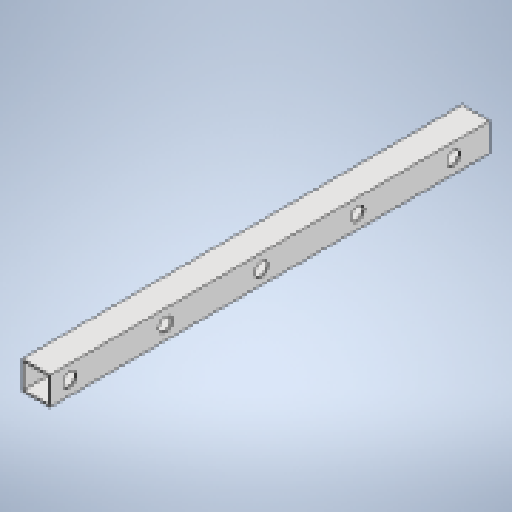
# Autodesk Inventor part: ANP 1434 FDS WAY tube4
Saved by Autodesk Inventor 2025.3 (Build 293356030, 356C)
## iProperties
Created: 2025-06-24
Part Number: ANP 1434 FDS WAY tube4
Material: Stainless Steel
Document SubType Name: Modeling
Designer: admin
Mass: 1762.25 g
Surface Area: 2283.33 cm^2
Volume: 220.281 cm^3
Density: 8 g/cm^3
Sheet Metal Rule: AISI304 2mm Die16
Sheet Metal Width: 0.000 mm
Sheet Metal Length: 0.000 mm
Sheet Metal Area: 0.000 mm^2
Appearance: Default
Stock Number: 30x30
Author: user
Autodesk Inventor part; units mm, degrees
ref_plane "YZ Plane" through (0, 0, 0) normal (1, 0, 0) x (0, 1, 0)
ref_plane "XZ Plane" through (0, 0, 0) normal (0, 1, 0) x (-1, 0, 0)
ref_plane "XY Plane" through (0, 0, 0) normal (0, 0, 1) x (1, 0, 0)
sketch "Sketch9" plane through (0, 0, 0) normal (0, 1, 0) x (-1, 0, 0)
  line L0 (17.5, 17.5) -> (-17.5, 17.5)
  line L1 (-17.5, 17.5) -> (-17.5, -17.5)
  line L2 (-17.5, -17.5) -> (17.5, -17.5)
  line L3 (17.5, -17.5) -> (17.5, 17.5)
  line L4 (17.5, 17.5) -> (-17.5, -17.5) construction
  line L5 (-17.5, 17.5) -> (17.5, -17.5) construction
  line L6 (-15.5, 15.5) -> (15.5, 15.5)
  line L7 (15.5, 15.5) -> (15.5, -15.5)
  line L8 (15.5, -15.5) -> (-15.5, -15.5)
  line L9 (-15.5, -15.5) -> (-15.5, 15.5)
  point P0 (0, 0)
  dimension "d172" = 35
  dimension "d173" = 35
  dimension "d174" = 2
  constraints: 20 end point, 4 parallel, 2 midpoint, 2 perpendicular, 1 horizontal, 3 other
  measures "d172" distance of L2.end L1.end
  measures "d173" distance of L0.end L1.end
  measures "d174" distance between parallel lines of L0 L6
extrude "Extrusion3" add sketch "Sketch9" against normal blind 550
sketch "Sketch10" plane through (0, 0, 0) normal (1, 0, 0) x (0, 1, 0)
  line L0 (0, 17.5) -> (0, -17.5) construction
  line L1 (0, 17.5) -> (-550, 17.5) construction
  line L2 (-550, -17.5) -> (-550, 17.5) construction
  line L3 (0, -17.5) -> (-550, -17.5) construction
  line L4 (-534, 8.5) -> (-517, 8.5)
  line L5 (-517, 8.5) -> (-517, -8.5)
  line L6 (-517, -8.5) -> (-534, -8.5)
  line L7 (-534, -8.5) -> (-534, 8.5)
  line L8 (-534, 8.5) -> (-517, -8.5) construction
  line L9 (-517, 8.5) -> (-534, -8.5) construction
  circle A0 centre (-525.5, 0) radius 8.5
  line L10 (0, 17.5) -> (0, -17.5) projected
  point P0 (0, 0)
  point P1 (0, 0)
  point P2 (-550, 0)
  dimension "d177" = 17
  dimension "d178" = 17
  dimension "d191" = 16
  constraints: 12 end point, 4 midpoint, 2 parallel, 1 centre point, 1 coincident, 1 horizontal, 1 horizontal alignment, 1 perpendicular, 1 tangent
  measures "d177" distance of L4.start L4.end
  measures "d178" distance of L4.end L5.end
  measures "d191" distance between parallel lines of L7 L2
extrude "Extrusion4" cut sketch "Sketch10" along normal through all contours A0
pattern_linear "Rectangular Pattern4" count 5 spacing 120 along (0, 1, 0) of "Extrusion4"
body "Solid4"
